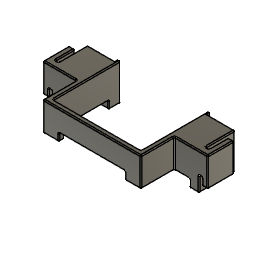
Nintendo 3DS - Dock holder v1.1 v23 (Autodesk Fusion 360 design; units mm, degrees)
Autodesk Fusion 360 part; units mm, degrees
sketch "Boceto1" plane through (0, 0, 0) normal (0, 0, 1) x (1, 0, 0)
  line L0 (-5.05, 0) -> (-5.05, 3.45)
  line L1 (-5.05, 3.45) -> (-8.5, 3.45)
  line L2 (-8.5, 3.45) -> (-8.5, 6.15)
  line L3 (-8.5, 6.15) -> (-7.6, 6.15)
  line L4 (-7.6, 6.15) -> (-7.6, 7.15)
  line L5 (-7.6, 7.15) -> (-4.8, 7.15)
  line L6 (-4.8, 7.15) -> (-4.8, 7.45)
  line L7 (-4.8, 7.45) -> (-4.5, 7.45)
  line L8 (-4.5, 7.45) -> (-4.5, 7.15)
  line L9 (-4.5, 7.15) -> (0, 7.15)
  line L10 (0, 0.55) -> (-4.5, 0.55)
  line L11 (-4.5, 0.55) -> (-4.5, 6.25)
  line L12 (0, 6.25) -> (-4.5, 6.25)
  line L13 (-5.05, 0) -> (0, 0)
  line L14 (0, 1.75) -> (0, 22.5)
  line L15 (5.05, 3.45) -> (8.5, 3.45)
  line L16 (4.8, 7.15) -> (4.8, 7.45)
  line L17 (7.6, 7.15) -> (4.8, 7.15)
  line L18 (4.5, 0.55) -> (4.5, 6.25)
  line L19 (5.05, 0) -> (0, 0)
  line L20 (0, 6.25) -> (4.5, 6.25)
  line L21 (5.05, 0) -> (5.05, 3.45)
  line L22 (0, 0.55) -> (4.5, 0.55)
  line L23 (8.5, 6.15) -> (7.6, 6.15)
  line L24 (4.8, 7.45) -> (4.5, 7.45)
  line L25 (4.5, 7.45) -> (4.5, 7.15)
  line L26 (7.6, 6.15) -> (7.6, 7.15)
  line L27 (8.5, 3.45) -> (8.5, 6.15)
  line L28 (4.5, 7.15) -> (0, 7.15)
  dimension "d2" = 3.45
  dimension "d3" = 2.7
  dimension "d4" = 0.9
  dimension "d5" = 1
  dimension "d6" = 2.8
  dimension "d7" = 0.3
  dimension "d8" = 0.3
  dimension "d9" = 0.3
  dimension "d10" = 4.5
  dimension "d11" = 3.45
  dimension "d13" = 0.55
  dimension "d14" = 0.55
  dimension "d15" = 0.9
  dimension "d16" = 5.05
  constraint perpendicular L0 L1
  constraint perpendicular L1 L2
  constraint perpendicular L2 L3
  constraint perpendicular L3 L4
  constraint perpendicular L4 L5
  constraint perpendicular L5 L6
  constraint perpendicular L6 L7
  constraint perpendicular L7 L8
  constraint perpendicular L8 L9
  constraint perpendicular L0 L10
  constraint perpendicular L11 L12
  constraint coincident L13.end L19.end
  constraint perpendicular L0 L13
  constraint symmetric L13.end L14 L19.end
  constraint symmetric L0.start L14 L19.start
  constraint symmetric L0.end L14 L15.start
  constraint symmetric L1.end L14 L15.end
  constraint symmetric L2.end L14 L23.start
  constraint symmetric L3.end L14 L23.end
  constraint symmetric L4.end L14 L17.start
  constraint symmetric L5.end L14 L16.start
  constraint symmetric L6.end L14 L16.end
  constraint symmetric L7.end L14 L24.end
  constraint symmetric L8.end L14 L25.end
  constraint symmetric L9.end L14 L28.end
  constraint symmetric L10.start L14 L22.start
  constraint symmetric L10.end L14 L18.start
  constraint symmetric L12.start L14 L20.start
  constraint symmetric L11.end L14 L18.end
  measures "d2" distance of L0.start L0.end
  measures "d3" distance of L1.end L2.end
  measures "d4" distance of L2.end L3.end
  measures "d5" distance of L3.end L4.end
  measures "d6" distance of L4.end L5.end
  measures "d7" distance of L5.end L6.end
  measures "d8" distance of L6.end L7.end
  measures "d9" distance of L7.end L8.end
  measures "d10" distance of L8.end L9.end
  measures "d11" distance of L0.end L1.end
  measures "d13" distance of L13.end L10.start
  measures "d14" horizontal distance of L0.end L10.end
  measures "d15" distance of L9.end L12.start
  measures "d16" distance of L13.end L0.start
extrude "Extruir1" add sketch "Boceto1" along normal blind 3.8
sketch "Boceto3" plane through (0, 0, 0) normal (0, 0, -1) x (1, 0, 0)
  line L0 (-4.5, -0.55) -> (4.5, -0.55)
  line L1 (4.5, -0.55) -> (4.5, -6.25)
  line L2 (4.5, -6.25) -> (-4.5, -6.25)
  line L3 (-4.5, -6.25) -> (-4.5, -0.55)
  line L4 (5.05, -3.45) -> (5.05, 0)
  line L5 (5.05, 0) -> (-5.05, 0)
  line L6 (-5.05, 0) -> (-5.05, -3.45)
  line L7 (-5.05, -3.45) -> (-8.5, -3.45)
  line L8 (-8.5, -3.45) -> (-8.5, -6.15)
  line L9 (-8.5, -6.15) -> (-7.6, -6.15)
  line L10 (-7.6, -6.15) -> (-7.6, -7.15)
  line L11 (-7.6, -7.15) -> (-4.8, -7.15)
  line L12 (-4.8, -7.15) -> (-4.8, -7.45)
  line L13 (-4.8, -7.45) -> (-4.5, -7.45)
  line L14 (-4.5, -7.45) -> (-4.5, -7.15)
  line L15 (-4.5, -7.15) -> (4.5, -7.15)
  line L16 (4.5, -7.15) -> (4.5, -7.45)
  line L17 (4.5, -7.45) -> (4.8, -7.45)
  line L18 (4.8, -7.45) -> (4.8, -7.15)
  line L19 (4.8, -7.15) -> (7.6, -7.15)
  line L20 (7.6, -7.15) -> (7.6, -6.15)
  line L21 (7.6, -6.15) -> (8.5, -6.15)
  line L22 (8.5, -6.15) -> (8.5, -3.45)
  line L23 (8.5, -3.45) -> (5.05, -3.45)
  line L24 (-7.6, -6.15) -> (-7.6, -3.45)
  line L25 (-6.604, -3.45) -> (-6.604, -6.25)
  line L26 (-4.5, -6.25) -> (-6.604, -6.25)
  line L27 (0, -1.75) -> (0, -22.5)
  line L28 (4.5, -6.25) -> (6.604, -6.25)
  line L29 (6.604, -3.45) -> (6.604, -6.25)
  line L30 (7.6, -6.15) -> (7.6, -3.45)
  line L31 (4.8, -7.15) -> (4.5, -7.15)
  line L32 (-4.8, -7.15) -> (-4.5, -7.15)
  dimension "d19" = 0.996
  constraint coincident L9.end L10.start
  constraint coincident L7 L24.end
  constraint perpendicular L7 L24
  constraint coincident L7 L25.start
  constraint perpendicular L7 L25
  constraint coincident L2.end L3.start
  constraint perpendicular L25 L26
  constraint symmetric L9.end L27 L20.end
  constraint symmetric L24.end L27 L30.end
  constraint symmetric L25.start L27 L29.start
  constraint symmetric L2.end L27 L1.end
  constraint symmetric L25.end L27 L28.end
  constraint coincident L18.end L19.start
  constraint coincident L15.end L16.start
  constraint symmetric L27 L18.end L11.end
  constraint symmetric L27 L15.end L14.end
  measures "d19" distance of L24.end L25.start
extrude "Extruir2" cut sketch "Boceto3" against normal blind 0.8 contours L0 L1 L3 L4 L5 L6 L7 L23 L25 L26 L28 L29 | L7 L8 L9 L24 | L21 L22 L23 L30
sketch "Boceto4" plane through (0, 0, 0.8) normal (0, 0, -1) x (1, 0, 0)
  line L0 (5.05, -3.45) -> (5.05, 0)
  line L1 (5.05, 0) -> (-5.05, 0)
  line L2 (-5.05, 0) -> (-5.05, -3.45)
  line L3 (-5.05, -3.45) -> (-6.604, -3.45)
  line L4 (-6.604, -3.45) -> (-6.604, -6.25)
  line L5 (-6.604, -6.25) -> (-4.5, -6.25)
  line L6 (-4.5, -6.25) -> (-4.5, -0.55)
  line L7 (-4.5, -0.55) -> (4.5, -0.55)
  line L8 (4.5, -0.55) -> (4.5, -6.25)
  line L9 (4.5, -6.25) -> (6.604, -6.25)
  line L10 (6.604, -6.25) -> (6.604, -3.45)
  line L11 (6.604, -3.45) -> (5.05, -3.45)
  line L12 (6.404, -6.05) -> (5.374, -6.05)
  line L13 (5.374, -6.05) -> (5.374, -3.65)
  line L14 (5.374, -3.65) -> (6.404, -3.65)
  line L15 (6.404, -3.65) -> (6.404, -6.05)
  line L16 (3.4, -0.55) -> (3.4, 0)
  line L17 (0, -1.75) -> (0, -22.5)
  line L18 (-6.404, -6.05) -> (-5.374, -6.05)
  line L19 (-6.404, -3.65) -> (-6.404, -6.05)
  line L20 (-5.374, -6.05) -> (-5.374, -3.65)
  line L21 (-5.374, -3.65) -> (-6.404, -3.65)
  line L22 (-3.4, -0.55) -> (-3.4, 0)
  dimension "d23" = 1.65
  dimension "d25" = 1.03
  dimension "d26" = 0.2
  dimension "d27" = 0.2
  dimension "d43" = 0.2
  constraint horizontal L12
  constraint vertical L13
  constraint horizontal L14
  constraint vertical L15
  constraint coincident L7 L16.start
  constraint coincident L1 L16.end
  constraint perpendicular L1 L16
  constraint symmetric L12.start L17 L18.start
  constraint symmetric L12.end L17 L18.end
  constraint symmetric L13.end L17 L20.end
  constraint symmetric L14.end L17 L19.start
  constraint symmetric L16.start L17 L22.start
  constraint symmetric L16.end L17 L22.end
  measures "d23" distance of L0.end L16.end
  measures "d25" distance of L12.start L12.end
  measures "d26" vertical distance of L0.start L13.end
  measures "d27" horizontal distance of L10.end L14.end
  measures "d43" vertical distance of L9.end L12.end
sketch "Boceto5" plane through (0, 0, 0.8) normal (0, 0, -1) x (1, 0, 0)
  line L0 (8.5, -6.15) -> (8.5, -3.45)
  line L1 (8.5, -3.45) -> (7.6, -3.45)
  line L2 (7.6, -3.45) -> (7.6, -6.15)
  line L3 (7.6, -6.15) -> (8.5, -6.15)
  line L4 (7.9, -6.15) -> (7.9, -3.45)
  dimension "d30" = 0.3
  constraint coincident L3 L4.start
  constraint coincident L1 L4.end
  constraint perpendicular L1 L4
  measures "d30" distance of L1.end L4.end
sketch "Boceto6" plane through (0, 0, 0.8) normal (0, 0, -1) x (1, 0, 0)
  line L0 (-7.6, -6.15) -> (-7.6, -3.45)
  line L1 (-7.6, -3.45) -> (-8.5, -3.45)
  line L2 (-8.5, -3.45) -> (-8.5, -6.15)
  line L3 (-8.5, -6.15) -> (-7.6, -6.15)
  line L4 (-7.9, -6.15) -> (-7.9, -3.45)
  dimension "d31" = 0.3
  constraint coincident L3 L4.start
  constraint coincident L1 L4.end
  constraint perpendicular L1 L4
  measures "d31" distance of L0.end L4.end
extrude "Extruir3" cut sketch "Boceto6" sketch "Boceto5" sketch "Boceto4" against normal blind 0.8 contours L0 L1 L3 L4 of sketch 2 contours L1 L2 L3 L4 of sketch 3 contours L1 L7 L16 L22 | L12 L13 L14 L15 | L18 L19 L20 L21
sketch "Boceto7" plane through (0, 0, 3.8) normal (0, 0, 1) x (-1, 0, 0)
  line L0 (-4.5, -0.55) -> (4.5, -0.55)
  line L1 (4.5, -0.55) -> (4.5, -6.25)
  line L2 (4.5, -6.25) -> (-4.5, -6.25)
  line L3 (-4.5, -6.25) -> (-4.5, -0.55)
  line L4 (-5.05, 0) -> (-5.05, -3.45)
  line L5 (-5.05, -3.45) -> (-8.5, -3.45)
  line L6 (-8.5, -3.45) -> (-8.5, -6.15)
  line L7 (-8.5, -6.15) -> (-7.6, -6.15)
  line L8 (-7.6, -6.15) -> (-7.6, -7.15)
  line L9 (-7.6, -7.15) -> (-4.8, -7.15)
  line L10 (-4.8, -7.15) -> (-4.8, -7.45)
  line L11 (-4.8, -7.45) -> (-4.5, -7.45)
  line L12 (-4.5, -7.45) -> (-4.5, -7.15)
  line L13 (-4.5, -7.15) -> (4.5, -7.15)
  line L14 (4.5, -7.15) -> (4.5, -7.45)
  line L15 (4.5, -7.45) -> (4.8, -7.45)
  line L16 (4.8, -7.45) -> (4.8, -7.15)
  line L17 (4.8, -7.15) -> (7.6, -7.15)
  line L18 (7.6, -7.15) -> (7.6, -6.15)
  line L19 (7.6, -6.15) -> (8.5, -6.15)
  line L20 (8.5, -6.15) -> (8.5, -3.45)
  line L21 (8.5, -3.45) -> (5.05, -3.45)
  line L22 (5.05, -3.45) -> (5.05, 0)
  line L23 (5.05, 0) -> (-5.05, 0)
  line L24 (-7.6, -6.15) -> (-7.6, -4.15)
  line L25 (-7.6, -4.15) -> (-7.9, -4.15)
  line L26 (-7.9, -4.15) -> (-7.9, -6.15)
  line L27 (-4.5, -6.25) -> (-4.5, -7.15)
  line L28 (0, -1.75) -> (0, -22.5)
  line L29 (7.9, -4.15) -> (7.9, -6.15)
  line L30 (7.6, -4.15) -> (7.9, -4.15)
  line L31 (7.6, -6.15) -> (7.6, -4.15)
  line L32 (4.5, -6.25) -> (4.5, -7.15)
  dimension "d32" = 2
  dimension "d33" = 0.3
  constraint coincident L7.end L8.start
  constraint perpendicular L7 L24
  constraint perpendicular L8 L25
  constraint coincident L7 L26.end
  constraint perpendicular L7 L26
  constraint coincident L2.end L3.start
  constraint coincident L12.end L13.start
  constraint symmetric L7.end L28 L18.end
  constraint symmetric L24.end L28 L30.start
  constraint symmetric L25.end L28 L29.start
  constraint symmetric L26.end L28 L29.end
  constraint symmetric L2.end L28 L1.end
  constraint symmetric L12.end L28 L13.end
  measures "d32" distance of L7.end L24.end
  measures "d33" distance of L24.end L25.end
extrude "Extruir4" cut sketch "Boceto7" against normal blind 1.3 contours L7 L24 L25 L26 | L19 L29 L30 L31
extrude "Extruir5" cut sketch "Boceto7" against normal blind 3.8 contours L2 L13 L27 L28 | L2 L13 L28 L32
fillet "Empalme2" radius 0.1 7 edges at (6.2, 7.15, 3.8) (7.6, 7.15, 1.9) (6.2, 7.15, 0) (-6.2, 7.15, 3.8) (-6.2, 7.15, 0) (-7.6, 7.15, 1.9) (5.374, 4.85, 1.6) 50 faces at (-4.5, 4.75, 2.8) (-8.3, 4.35, 0.8) (-1.1333, 0.55, 3.0667) (-1.1333, 0, 3.0667) (7.6, 5.5833, 0.5333) (7.7, 4.35, 1.6) (-5.8167, 4.9167, 3.8) (-1.1333, 0.1833, 1.6) (-7.268, 5.6167, 0) (8.5, 4.35, 1.8) (-5.0827, 5.3167, 0.8) (-5.7173, 3.65, 1.0667) (5.7173, 3.65, 1.0667) (4.7, 7.45, 1.2667) (-7.9, 4.8167, 3.3667) (6.404, 4.45, 1.0667) (6.0607, 5.25, 1.6) (-5.7173, 5.25, 1.6) (-5.374, 5.25, 1.0667) (-6.404, 4.45, 1.0667) (5.374, 5.25, 1.0667) (-8.3, 6.15, 2.3667) (-7.7, 4.8167, 2.5) (-5.05, 1.15, 1.8) (-3.4, 0.3667, 1.0667) (5.05, 1.15, 1.8) (6.0607, 6.05, 1.0667) (7.05, 3.45, 3.0667) (3.4, 0.3667, 1.0667) (-7.7, 4.15, 3.3667) (-8.5, 5.25, 2.8) (7.7, 4.15, 3.3667) (-6.0607, 6.05, 1.0667) (7.7, 5.4833, 2.5) (-4.7, 7.45, 1.2667) (7.9, 4.8167, 3.3667) (8.3, 6.15, 2.3667) (-5.9027, 6.25, 0.5333) (7.9, 5.25, 1.0667) (7.268, 5.6167, 0) (-7.05, 3.45, 3.0667) (-6.604, 4.3833, 0.2667) (-7.6, 5.5833, 0.5333) (8.1, 4.35, 0.8) (4.5, 4.75, 2.8) (-7.9, 5.25, 1.0667) (-7.7, 5.25, 1.6) (5.2013, 6.25, 0.5333) (5.0827, 5.3167, 0.8) (6.604, 4.3833, 0.2667)
delete_face "SuprimirCaras1" 6 faces at (6.5498, 4.4167, 0.7889) (6.5171, 6.2328, 0.7546) (5.2347, 6.2, 0.7866) (-5.2347, 6.2, 0.7866) (-6.5171, 6.2328, 0.7546) (-6.5498, 4.4167, 0.7889)
equation "d31 = d30"
